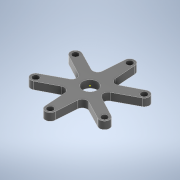
# Autodesk Inventor part: Extension
Saved by Autodesk Inventor 2021 (Build 250183000, 183)
## iProperties
Created: 2021-04-02
Part Number: Extension
Material: Genérico
Document SubType Name: Modeling
Designer: diego
Density: 1 g/cm^3
Appearance: Suave - Negro
Author: diego
Autodesk Inventor part; units mm, degrees
ref_plane "YZ Plane" through (0, 0, 0) normal (1, 0, 0) x (0, 1, 0)
ref_plane "XZ Plane" through (0, 0, 0) normal (0, 1, 0) x (-1, 0, 0)
ref_plane "XY Plane" through (0, 0, 0) normal (0, 0, 1) x (1, 0, 0)
sketch "Boceto1" plane through (0, 0, 0) normal (0, 1, 0) x (-1, 0, 0)
  circle A0 centre (0, -16) radius 2
  circle A1 centre (13.856406, -8) radius 2
  circle A2 centre (13.856406, 8) radius 2
  circle A3 centre (0, 16) radius 2
  circle A4 centre (-13.856406, 8) radius 2
  circle A5 centre (-13.856406, -8) radius 2
  line L0 (-12.759095, -9.672097) -> (-5.490746, -5.928235)
  line L1 (-6.410449, -1.764863) -> (-14.746933, -6.209201)
  line L2 (-6.410449, 1.764863) -> (-14.746933, 6.209201)
  line L3 (-12.759095, 9.672097) -> (-5.490746, 5.928235)
  line L4 (2, 16) -> (2.583184, 7.574131)
  line L5 (-2, 16) -> (-2.579628, 7.569051)
  line L6 (2.579349, -7.573106) -> (2, -16)
  line L7 (-2.579628, -7.569051) -> (-2, -16)
  line L8 (12.856406, 9.732051) -> (5.495313, 5.934789)
  line L9 (14.856406, 6.267949) -> (6.4102, 1.764839)
  line L10 (14.856406, -6.267949) -> (6.4102, -1.764839)
  line L11 (12.856406, -9.732051) -> (5.491541, -5.932843)
  circle A6 centre (0, 0) radius 3
  arc A7 (-6.410449, -1.764863) -> (-6.410449, 1.764863) centre (-7.351331, 0) ccw
  arc A8 (-2.579628, -7.569051) -> (-5.490746, -5.928235) centre (-4.574918, -7.706228) ccw
  arc A9 (5.491541, -5.932843) -> (2.579349, -7.573106) centre (4.574639, -7.710282) ccw
  arc A10 (6.4102, 1.764839) -> (6.4102, -1.764839) centre (7.351127, 0) ccw
  arc A11 (2.583184, 7.574131) -> (5.495313, 5.934789) centre (4.578411, 7.712228) ccw
  arc A12 (-5.490746, 5.928235) -> (-2.579628, 7.569051) centre (-4.574918, 7.706228) ccw
  point P0 (0, -3.1)
  point P1 (-3.1, 0)
  point P2 (0, 3.1)
  point P3 (3.1, 0)
  dimension "d17" = 360
  dimension "d19" = 6
  dimension "d20" = 2
  constraints: 24 end point, 24 point on circle, 13 centre point, 12 tangent, 11 point on line, 5 equal radius, 3 coincident, 1 parallel, 17 other
  measures "d19" diameter of A6
  measures "d20" radius of A7
sketch "Boceto1 outline for Extrusión1" plane through (0, 0, 0) normal (0, 1, 0) x (-1, 0, 0)
  arc A0 (5.495313, 5.934789) -> (2.583184, 7.574131) centre (4.578411, 7.712228) cw
  line L0 (12.856406, 9.732051) -> (5.495313, 5.934789)
  line L1 (2.583184, 7.574131) -> (2, 16)
  arc A1 (14.856406, 6.267949) -> (12.856406, 9.732051) centre (13.856406, 8) ccw
  arc A2 (2, 16) -> (-2, 16) centre (0, 16) ccw
  line L2 (6.4102, 1.764839) -> (14.856406, 6.267949)
  line L3 (-2, 16) -> (-2.579628, 7.569051)
  arc A3 (6.4102, -1.764839) -> (6.4102, 1.764839) centre (7.351127, 0) cw
  arc A4 (-2.579628, 7.569051) -> (-5.490746, 5.928235) centre (-4.574918, 7.706228) cw
  line L4 (14.856406, -6.267949) -> (6.4102, -1.764839)
  line L5 (-5.490746, 5.928235) -> (-12.759095, 9.672097)
  arc A5 (12.856406, -9.732051) -> (14.856406, -6.267949) centre (13.856406, -8) ccw
  arc A6 (-12.759095, 9.672097) -> (-14.746933, 6.209201) centre (-13.856406, 8) ccw
  line L6 (5.491541, -5.932843) -> (12.856406, -9.732051)
  line L7 (-14.746933, 6.209201) -> (-6.410449, 1.764863)
  arc A7 (2.579349, -7.573106) -> (5.491541, -5.932843) centre (4.574639, -7.710282) cw
  arc A8 (-6.410449, 1.764863) -> (-6.410449, -1.764863) centre (-7.351331, 0) cw
  line L8 (2, -16) -> (2.579349, -7.573106)
  line L9 (-6.410449, -1.764863) -> (-14.746933, -6.209201)
  arc A9 (-2, -16) -> (2, -16) centre (0, -16) ccw
  arc A10 (-14.746933, -6.209201) -> (-12.759095, -9.672097) centre (-13.856406, -8) ccw
  line L10 (-2.579628, -7.569051) -> (-2, -16)
  line L11 (-12.759095, -9.672097) -> (-5.490746, -5.928235)
  arc A11 (-5.490746, -5.928235) -> (-2.579628, -7.569051) centre (-4.574918, -7.706228) cw
  circle A12 centre (0, 0) radius 3
extrude "Extrusión1" add sketch "Boceto1 outline for Extrusión1" along normal blind 3
sketch "Boceto2" plane through (0, 3, 0) normal (0, 1, 0) x (1, 0, 0)
  arc A0 (-14.856406, -6.267949) -> (-12.856406, -9.732051) centre (-13.856406, -8) ccw
  circle A1 centre (-13.856406, -8) radius 1.25
  arc A2 (-2, -16) -> (2, -16) centre (0, -16) ccw
  circle A3 centre (0, -16) radius 1.25
  arc A4 (-12.856406, 9.732051) -> (-14.856406, 6.267949) centre (-13.856406, 8) ccw
  circle A5 centre (-13.856406, 8) radius 1.25
  arc A6 (2, 16) -> (-2, 16) centre (0, 16) ccw
  circle A7 centre (0, 16) radius 1.25
  arc A8 (14.746933, 6.209201) -> (12.759095, 9.672097) centre (13.856406, 8) ccw
  circle A9 centre (13.856406, 8) radius 1.25
  arc A10 (12.759095, -9.672097) -> (14.746933, -6.209201) centre (13.856406, -8) ccw
  circle A11 centre (13.856406, -8) radius 1.25
  point P0 (0, 0)
  dimension "d23" = 2.5
  dimension "d24" = 2.5
  dimension "d25" = 2.5
  dimension "d26" = 2.5
  dimension "d27" = 2.5
  dimension "d28" = 2.5
  constraints: 6 centre point, 6 coincident
  measures "d23" diameter of A1
  measures "d24" diameter of A3
  measures "d25" diameter of A5
  measures "d26" diameter of A7
  measures "d27" diameter of A9
  measures "d28" diameter of A11
hole "Agujero1" at (0, 3, -16) at (-13.856406, 3, -8) at (0, 3, 16) at (13.856406, 3, 8) at (13.856406, 3, -8) direction (0, -1, 0) diameter 2.5 end through all
sketch "Boceto3" plane through (0, 3, 0) normal (0, 1, 0) x (1, 0, 0)
  arc A0 (-14.856406, -6.267949) -> (-12.856406, -9.732051) centre (-13.856406, -8) ccw
  circle A1 centre (-13.856406, -8) radius 1.25
  point P0 (0, 0)
  dimension "d36" = 2.5
  constraints: 1 centre point, 1 coincident
  measures "d36" diameter of A1
hole "Agujero2" at (-13.856406, 3, 8) direction (0, -1, 0) diameter 2.5 end through all
sketch "Boceto4" plane through (0, 3, 0) normal (0, 1, 0) x (1, 0, 0)
  point P0 (0, 0)
